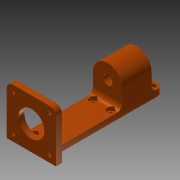
# Autodesk Inventor part: xy mount
Saved by Autodesk Inventor 2013 (Build 170138000, 138)
## iProperties
Created: 2013-07-22
Part Number: xy mount
Material: Generic
Document SubType Name: Modeling
Designer: employee
Density: 1 g/cm^3
Mass: 33.2296 g
Surface Area: 129.182 cm^2
Volume: 33.2296 cm^3
Author: employee
Autodesk Inventor part; units mm, degrees
ref_plane "YZ Plane" through (0, 0, 0) normal (1, 0, 0) x (0, 1, 0)
ref_plane "XZ Plane" through (0, 0, 0) normal (0, 1, 0) x (-1, 0, 0)
ref_plane "XY Plane" through (0, 0, 0) normal (0, 0, 1) x (1, 0, 0)
sketch "Sketch1" plane through (0, 0, 0) normal (0, 1, 0) x (-1, 0, 0)
  line L0 (-21, 42) -> (21, 42)
  line L1 (21, 42) -> (21, 0)
  line L2 (21, 0) -> (-21, 0)
  line L3 (-21, 0) -> (-21, 42)
  point P0 (0, 0)
  point P1 (0, 0)
  dimension "d0" = 42
  constraints: 8 end point, 2 parallel, 2 perpendicular, 1 coincident, 1 horizontal, 1 midpoint
  measures "d0" distance of L2.end L0.start
extrude "Extrusion1" add sketch "Sketch1" along normal blind 5
sketch "Sketch2" plane through (0, 5, 0) normal (0, 1, 0) x (1, 0, 0)
  line L0 (-21, -42) -> (21, -42) projected
  line L1 (-21, 0) -> (-21, -42) projected
  circle A0 centre (0, -21) radius 11.05
  line L2 (15.5, -36.5) -> (-15.5, -36.5)
  line L3 (-15.5, -36.5) -> (-15.5, -5.5)
  line L4 (-15.5, -5.5) -> (15.5, -5.5)
  line L5 (15.5, -5.5) -> (15.5, -36.5)
  circle A1 centre (15.5, -36.5) radius 1.55
  circle A2 centre (-15.5, -36.5) radius 1.55
  circle A3 centre (-15.5, -5.5) radius 1.55
  circle A4 centre (15.5, -5.5) radius 1.55
  point P0 (0, 0)
  point P1 (-21, -21)
  point P2 (0, -42)
  dimension "d4" = 31
  dimension "d5" = 22.1
  dimension "d6" = 3.1
  constraints: 8 end point, 5 centre point, 5 coincident, 3 equal radius, 2 midpoint, 1 horizontal, 1 horizontal alignment, 1 vertical alignment, 9 other
  measures "d4" distance of L2.start L2.end
  measures "d5" diameter of A0
  measures "d6" diameter of A1
extrude "Extrusion2" cut sketch "Sketch2" against normal through all contours A0 | A2 L3 L2 | L2 L3 A2 | A1 L5 L2 | L2 L5 A1 | A3 L4 L3 | L3 L4 A3 | A4 L4 L5 | L5 L4 A4
sketch "Sketch3" plane through (0, 5, 0) normal (0, 1, 0) x (1, 0, 0)
  line L0 (21, 0) -> (-21, 0) projected
  line L1 (12.5, -5) -> (-12.5, -5)
  line L2 (-12.5, -5) -> (-12.5, 0)
  line L3 (-12.5, 0) -> (12.5, 0)
  line L4 (12.5, 0) -> (12.5, -5)
  point P0 (0, 0)
  point P1 (0, 0)
  dimension "d9" = 25
  dimension "d11" = 5
  constraints: 8 end point, 2 midpoint, 2 parallel, 1 horizontal, 1 perpendicular
  measures "d9" distance of L1.start L1.end
  measures "d11" distance of L1.end L2.end
extrude "Extrusion3" add sketch "Sketch3" along normal blind 60
sketch "Sketch7" plane through (0, 0, 0) normal (0, -1, 0) x (1, 0, 0)
  circle A0 centre (0, 21) radius 11.05 projected
  point P0 (0, 0)
extrude "Extrusion7" cut sketch "Sketch7" against normal through all
sketch "Sketch8" plane through (0, 65, 0) normal (0, 1, 0) x (1, 0, 0)
  line L0 (12.5, 0) -> (-12.5, 0) projected
  line L1 (-12.5, 0) -> (-12.5, -5) projected
  line L2 (-12.5, -5) -> (12.5, -5) projected
  line L3 (12.5, -5) -> (12.5, 0) projected
  circle A0 centre (0, -21) radius 11.05 projected
  circle A1 centre (-15.5, -5.5) radius 1.55 projected
  circle A2 centre (15.5, -36.5) radius 1.55 projected
  circle A3 centre (-15.5, -36.5) radius 1.55 projected
  circle A4 centre (15.5, -5.5) radius 1.55 projected
  line L4 (21, -42) -> (-21, -42) projected
  line L5 (-21, -42) -> (-21, 0) projected
  line L6 (-21, 0) -> (21, 0) projected
  line L7 (21, 0) -> (21, -42) projected
  line L8 (-12.5, -5) -> (-12.5, -21)
  arc A5 (-12.5, -21) -> (12.5, -21) centre (0, -21) ccw
  line L9 (12.5, -21) -> (12.5, -5)
  circle A6 centre (0, -21) radius 4.05
  point P0 (0, 0)
  dimension "d25" = 8.1
  constraints: 4 end point, 2 centre point, 2 point on circle, 2 tangent, 1 coincident, 1 collinear, 1 concentric, 1 parallel
  measures "d25" diameter of A6
extrude "Extrusion8" add sketch "Sketch8" along normal blind 25 contours L3 L2 L1 L0 | L9 A5 L8 L2 | A0
sketch "Sketch9" plane through (0, 90, 0) normal (0, 1, 0) x (1, 0, 0)
  line L0 (12.5, 0) -> (-12.5, 0) projected
  line L1 (-12.5, 0) -> (-12.5, -21) projected
  line L2 (12.5, -21) -> (12.5, 0) projected
  line L3 (-12.5, -5) -> (12.5, -5) projected
  point P0 (0, 0)
extrude "Extrusion9" add sketch "Sketch9" along normal blind 10
sketch "Sketch10" plane through (21, 0, 0) normal (0, 0, -1) x (-1, 0, 0)
  line L0 (33.5, 5) -> (42, 5) projected
  line L1 (33.5, 5) -> (33.5, 100) projected
  line L2 (33.5, 65) -> (8.5, 65) projected
  line L3 (8.5, 65) -> (8.5, 90) projected
  line L4 (33.5, 90) -> (8.5, 90) projected
  line L5 (33.5, 65) -> (33.5, 90) projected
  line L6 (0, 0) -> (42, 0) projected
  line L7 (0, 0) -> (0, 5) projected
  line L8 (42, 5) -> (0, 5) projected
  line L9 (42, 0) -> (42, 5) projected
  line L10 (28.5, 95) -> (13.5, 95)
  line L11 (13.5, 95) -> (13.5, 60)
  line L12 (13.5, 60) -> (28.5, 60)
  line L13 (28.5, 60) -> (28.5, 95)
  line L14 (28.5, 60) -> (13.5, 60)
  line L15 (13.5, 60) -> (13.5, 10)
  line L16 (13.5, 10) -> (28.5, 10)
  line L17 (28.5, 10) -> (28.5, 60)
  line L18 (33.5, 65) -> (33.5, 5)
  circle A0 centre (28.5, 95) radius 1.55
  circle A1 centre (13.5, 95) radius 1.55
  circle A2 centre (13.5, 60) radius 1.55
  circle A3 centre (28.5, 60) radius 1.55
  circle A4 centre (28.5, 10) radius 1.55
  circle A5 centre (13.5, 10) radius 1.55
  point P0 (21, 0)
  point P1 (21, 95)
  point P2 (21, 90)
  point P3 (28.5, 77.5)
  point P4 (33.5, 77.5)
  point P5 (28.5, 35)
  point P6 (33.5, 35)
  dimension "d31" = 5
  dimension "d32" = 5
  dimension "d33" = 3.1
  constraints: 18 end point, 6 centre point, 6 coincident, 6 midpoint, 5 equal radius, 4 parallel, 3 perpendicular, 2 horizontal, 2 horizontal alignment, 1 vertical alignment
  measures "d31" distance between parallel lines of L2 L14
  measures "d32" distance between parallel lines of L1 L13
  measures "d33" diameter of A4
extrude "Extrusion10" cut sketch "Sketch10" against normal blind 2.5 contours A3 L17 L13 | L13 L12 A3 | A0 L10 L13 | L13 L10 A0 | A2 L12 L11 | L11 L15 A2 | L17 A3 L12 | A1 L10 L11 | L11 L10 A1 | L12 A2 L15 | A5 L16 L15 | L15 L16 A5 | A4 L16 L17 | L17 L16 A4
sketch "Sketch11" plane through (-7.5, 95, 2.5) normal (0, 0, -1) x (-1, 0, 0)
  circle A0 centre (-15, -85) radius 1.55 projected
  circle A1 centre (0, -35) radius 1.55 projected
  circle A2 centre (-15, 0) radius 1.55 projected
  circle A3 centre (0, 0) radius 1.55 projected
  circle A4 centre (-15, -35) radius 1.55 projected
  circle A5 centre (0, -85) radius 1.55 projected
  line L0 (-28.5, -95) -> (-28.5, -90) projected
  line L1 (-28.5, -90) -> (-20, -90) projected
  line L2 (-20, -90) -> (-20, 5) projected
  line L3 (-20, 5) -> (5, 5) projected
  line L4 (5, 5) -> (5, -90) projected
  line L5 (5, -90) -> (13.5, -90) projected
  line L6 (13.5, -90) -> (13.5, -95) projected
  line L7 (13.5, -95) -> (-28.5, -95) projected
  line L8 (-15, -81.7668) -> (-12.2, -83.3834)
  line L9 (-12.2, -83.3834) -> (-12.2, -86.6166)
  line L10 (-12.2, -86.6166) -> (-15, -88.2332)
  line L11 (-15, -88.2332) -> (-17.8, -86.6166)
  line L12 (-17.8, -86.6166) -> (-17.8, -83.3834)
  line L13 (-17.8, -83.3834) -> (-15, -81.7668)
  line L14 (0, -81.7668) -> (2.8, -83.3834)
  line L15 (2.8, -83.3834) -> (2.8, -86.6166)
  line L16 (2.8, -86.6166) -> (0, -88.2332)
  line L17 (0, -88.2332) -> (-2.8, -86.6166)
  line L18 (-2.8, -86.6166) -> (-2.8, -83.3834)
  line L19 (-2.8, -83.3834) -> (0, -81.7668)
  line L20 (-15, -31.7668) -> (-12.2, -33.3834)
  line L21 (-12.2, -33.3834) -> (-12.2, -36.6166)
  line L22 (-12.2, -36.6166) -> (-15, -38.2332)
  line L23 (-15, -38.2332) -> (-17.8, -36.6166)
  line L24 (-17.8, -36.6166) -> (-17.8, -33.3834)
  line L25 (-17.8, -33.3834) -> (-15, -31.7668)
  line L26 (0, -31.7668) -> (2.8, -33.3834)
  line L27 (2.8, -33.3834) -> (2.8, -36.6166)
  line L28 (2.8, -36.6166) -> (0, -38.2332)
  line L29 (0, -38.2332) -> (-2.8, -36.6166)
  line L30 (-2.8, -36.6166) -> (-2.8, -33.3834)
  line L31 (-2.8, -33.3834) -> (0, -31.7668)
  line L32 (-15, 3.2332) -> (-12.2, 1.6166)
  line L33 (-12.2, 1.6166) -> (-12.2, -1.6166)
  line L34 (-12.2, -1.6166) -> (-15, -3.2332)
  line L35 (-15, -3.2332) -> (-17.8, -1.6166)
  line L36 (-17.8, -1.6166) -> (-17.8, 1.6166)
  line L37 (-17.8, 1.6166) -> (-15, 3.2332)
  line L38 (0, 3.2332) -> (2.8, 1.6166)
  line L39 (2.8, 1.6166) -> (2.8, -1.6166)
  line L40 (2.8, -1.6166) -> (0, -3.2332)
  line L41 (0, -3.2332) -> (-2.8, -1.6166)
  line L42 (-2.8, -1.6166) -> (-2.8, 1.6166)
  line L43 (-2.8, 1.6166) -> (0, 3.2332)
  point P0 (-7.5, -95)
  dimension "d36" = 5.6
  constraints: 72 end point, 6 coincident, 5 equal length, 5 vertical, 1 vertical alignment, 78 other
  measures "d36" distance between parallel lines of L33 L36
extrude "Extrusion11" cut sketch "Sketch11" against normal through all contours A0 | A1 | A2 | A3 | A4 | A5 | L8 L9 L10 L11 L12 L13 | L14 L15 L16 L17 L18 L19 | L20 L21 L22 L23 L24 L25 | L26 L27 L28 L29 L30 L31 | L32 L33 L34 L35 L36 L37 | L38 L39 L40 L41 L42 L43
fillet "Fillet1" radius 5 5 edges at (0, 90, 5) (0, 65, 5) (-21, 2.5, 42) (21, 2.5, 42) (0, 5, 5)
fillet "Fillet2" radius 5 2 edges at (-12.5, 100, 2.5) (12.5, 100, 2.5)
body "Solid1"
